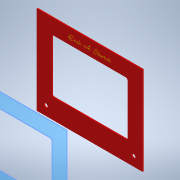
# Autodesk Inventor part: front
Saved by Autodesk Inventor 2022 (Build 260153000, 153)
## iProperties
Created: 2023-08-31
Part Number: front
Material: Generic
Document SubType Name: Modeling
Designer: THK
Density: 1 g/cm^3
Appearance: Red
Author: THK
Autodesk Inventor part; units mm, degrees
ref_plane "YZ Plane" through (0, 0, 0) normal (1, 0, 0) x (0, 1, 0)
ref_plane "XZ Plane" through (0, 0, 0) normal (0, 1, 0) x (-1, 0, 0)
ref_plane "XY Plane" through (0, 0, 0) normal (0, 0, 1) x (1, 0, 0)
sketch "Sketch1" plane through (0, 0, 0) normal (0, 0, 1) x (1, 0, 0)
  line L0 (-264.1156, 220.8859) -> (264.1156, 220.8859)
  line L1 (264.1156, 220.8859) -> (264.1156, -220.8859)
  line L2 (264.1156, -220.8859) -> (-264.1156, -220.8859)
  line L3 (-264.1156, -220.8859) -> (-264.1156, 220.8859)
  line L4 (-264.1156, 220.8859) -> (264.1156, -220.8859) construction
  line L5 (264.1156, 220.8859) -> (-264.1156, -220.8859) construction
  point P0 (0, 0)
  dimension "d0" = 528.2313
  dimension "d1" = 441.7719
  constraints: 12 end point, 2 midpoint, 2 parallel, 1 horizontal, 1 perpendicular
  measures "d0" distance of L1.end L2.end
  measures "d1" distance of L0.end L1.end
extrude "Extrusion1" add sketch "Sketch1" against normal blind 6
sketch "Sketch2" plane through (0, 0, 0) normal (0, 0, 1) x (1, 0, 0)
  line L0 (-181.2094, 146.2703) -> (181.2094, 146.2703)
  line L1 (189.5, 137.9797) -> (189.5, -113.1078)
  line L2 (181.2094, -121.3984) -> (-181.2094, -121.3984)
  line L3 (-189.5, -113.1078) -> (-189.5, 137.9797)
  line L4 (-189.5, 146.2703) -> (189.5, -121.3984) construction
  line L5 (189.5, 146.2703) -> (-189.5, -121.3984) construction
  line L6 (189.5, 105.3059) -> (264.1156, 105.3059) construction
  line L7 (264.1156, 220.8859) -> (264.1156, -220.8859) projected
  line L8 (72.6661, 146.2703) -> (72.6661, 220.8859) construction
  line L9 (-264.1156, 220.8859) -> (264.1156, 220.8859) projected
  arc A0 (-181.2094, 146.2703) -> (-189.5, 137.9797) centre (-181.2094, 137.9797) ccw
  arc A1 (189.5, 137.9797) -> (181.2094, 146.2703) centre (181.2094, 137.9797) ccw
  arc A2 (181.2094, -121.3984) -> (189.5, -113.1078) centre (181.2094, -113.1078) ccw
  arc A3 (-189.5, -113.1078) -> (-181.2094, -121.3984) centre (-181.2094, -113.1078) ccw
  point P0 (0, 0)
  point P1 (0, 12.4359)
  point P2 (0, 12.4359)
  dimension "d4" = 267.6687
  dimension "d5" = 379
  dimension "d6" = 74.6156
  dimension "d7" = 8.2906
  constraints: 16 end point, 12 point on line, 8 point on circle, 8 tangent, 4 centre point, 3 equal radius, 3 midpoint, 2 horizontal, 2 parallel, 2 perpendicular, 1 vertical, 1 vertical alignment
  measures "d4" distance between parallel lines of L2 L0
  measures "d5" distance between parallel lines of L1 L3
  measures "d6" distance between parallel lines of L7 L1
  measures "d7" radius of A0
extrude "Extrusion2" cut sketch "Sketch2" against normal through all
sketch "Sketch3" plane through (0, 0, 0) normal (0, 0, 1) x (1, 0, 0)
  line L0 (-264.1156, -220.8859) -> (-264.1156, 220.8859) construction
  line L1 (-264.1156, -220.8859) -> (-219.1094, -220.8859) construction
  line L2 (-219.1094, -220.8859) -> (-219.1094, -175.8797) construction
  line L3 (-219.1094, -175.8797) -> (-264.1156, -175.8797) construction
  line L4 (-264.1156, -175.8797) -> (-264.1156, -220.8859) construction
  point P0 (0, 0)
  dimension "d10" = 45.0063
  dimension "d11" = 45.0063
  constraints: 8 end point, 2 parallel, 1 coincident, 1 horizontal, 1 perpendicular
  measures "d10" distance of L3.end L2.end
  measures "d11" distance of L2.end L1.end
hole "Hole1" at (-219.1094, -175.8797, 0) direction (0, 0, -1) diameter 19 end through all
mirror "Mirror1" about plane through (0, 0, 0) normal (1, 0, 0) of "Hole1"
sketch "Sketch4" plane through (0, 0, 0) normal (0, 0, 1) x (1, 0, 0)
  line L0 (-128.1015, 195.1507) -> (128.1015, 195.1507) construction
  line L1 (128.1015, 195.1507) -> (128.1015, 162.8739) construction
  line L2 (128.1015, 162.8739) -> (-128.1015, 162.8739) construction
  line L3 (-128.1015, 162.8739) -> (-128.1015, 195.1507) construction
  line L4 (-189.5, 185.6016) -> (189.5, 185.6016) projected
  line L5 (-189.5, -121.3984) -> (-189.5, 185.6016) projected
  line L6 (189.5, -121.3984) -> (-189.5, -121.3984) projected
  line L7 (189.5, 185.6016) -> (189.5, -121.3984) projected
  spline S0 degree 2 poles (-100.767, 183.5729) (-99.0504, 183.5729) (-92.1658, 183.3172) (-90.4492, 183.3172) knots 0 0 0 1 2 2 2
  spline S1 degree 2 poles (-90.4492, 183.3172) (-87.7831, 183.3172) (-86.8335, 183.445) knots 0 0 0 1 1 1
  spline S2 degree 2 poles (-86.8335, 183.445) (-84.7699, 183.7372) (-83.5829, 184.8329) knots 0 0 0 1 1 1
  spline S3 degree 2 poles (-83.5829, 184.8329) (-84.3316, 182.2398) (-87.363, 180.8519) knots 0 0 0 1 1 1
  spline S4 degree 2 poles (-87.363, 180.8519) (-88.5866, 180.2858) (-90.5223, 180.2858) knots 0 0 0 1 1 1
  spline S5 degree 2 poles (-90.5223, 180.2858) (-90.924, 180.2858) (-94.1381, 180.3589) knots 0 0 0 1 1 1
  line L8 (-94.1381, 180.3589) -> (-97.7721, 180.3589)
  spline S6 degree 2 poles (-97.7721, 180.3589) (-98.2286, 180.3589) (-99.9452, 180.2858) knots 0 0 0 1 1 1
  spline S7 degree 2 poles (-99.9452, 180.2858) (-99.7809, 179.2084) (-98.5573, 177.784) knots 0 0 0 1 1 1
  spline S8 degree 2 poles (-98.5573, 177.784) (-96.7129, 175.6291) (-91.0884, 173.0725) (-88.1848, 173.0725) knots 0 0 0 1 2 2 2
  spline S9 degree 2 poles (-88.1848, 173.0725) (-85.9752, 173.0725) (-80.4237, 174.8621) (-78.7619, 176.1404) knots 0 0 0 1 2 2 2
  spline S10 degree 2 poles (-78.7619, 176.1404) (-79.328, 175.0265) (-80.6063, 173.9308) knots 0 0 0 1 1 1
  spline S11 degree 2 poles (-80.6063, 173.9308) (-82.615, 172.2507) (-88.0935, 170.2785) (-90.7779, 170.2785) knots 0 0 0 1 2 2 2
  spline S12 degree 2 poles (-90.7779, 170.2785) (-92.7319, 170.2785) (-97.4069, 171.7942) (-98.8861, 172.9812) knots 0 0 0 1 2 2 2
  spline S13 degree 2 poles (-98.8861, 172.9812) (-100.4931, 174.2595) (-102.8123, 178.3136) (-103.141, 180.3954) knots 0 0 0 1 2 2 2
  spline S14 degree 2 poles (-103.141, 180.3954) (-104.748, 180.3223) (-105.3141, 180.2858) knots 0 0 0 1 1 1
  spline S15 degree 2 poles (-105.3141, 180.2858) (-106.4646, 180.1945) (-107.4142, 179.8658) knots 0 0 0 1 1 1
  spline S16 degree 2 poles (-107.4142, 179.8658) (-106.0993, 182.7328) (-102.8305, 183.4816) knots 0 0 0 1 1 1
  spline S17 degree 2 poles (-102.8305, 183.4816) (-101.8079, 188.3026) (-98.6852, 191.0053) knots 0 0 0 1 1 1
  spline S18 degree 2 poles (-98.6852, 191.0053) (-96.4573, 192.941) (-90.2849, 195.1507) (-87.2717, 195.1507) knots 0 0 0 1 2 2 2
  spline S19 degree 2 poles (-87.2717, 195.1507) (-84.2403, 195.1507) (-81.8298, 194.2559) knots 0 0 0 1 1 1
  spline S20 degree 2 poles (-81.8298, 194.2559) (-78.4697, 193.0506) (-78.4697, 190.5122) knots 0 0 0 1 1 1
  spline S21 degree 2 poles (-78.4697, 190.5122) (-78.4697, 188.4304) (-80.4237, 185.7277) knots 0 0 0 1 1 1
  spline S22 degree 2 poles (-80.4237, 185.7277) (-80.3506, 188.1383) (-82.4872, 190.8957) (-84.8612, 191.6627) knots 0 0 0 1 2 2 2
  spline S23 degree 2 poles (-84.8612, 191.6627) (-86.943, 192.3201) (-89.2805, 192.3201) knots 0 0 0 1 1 1
  spline S24 degree 2 poles (-89.2805, 192.3201) (-91.8736, 192.3201) (-94.7042, 191.3705) knots 0 0 0 1 1 1
  spline S25 degree 2 poles (-94.7042, 191.3705) (-97.8634, 190.3114) (-100.5661, 186.8417) (-100.767, 183.5729) knots 0 0 0 1 2 2 2
  line L9 (-74.2148, 185.9651) -> (-71.7129, 186.4217)
  line L10 (-71.7129, 186.4217) -> (-72.4434, 182.532)
  spline S26 degree 2 poles (-72.4434, 182.532) (-72.3703, 182.532) (-72.1147, 182.532) knots 0 0 0 1 1 1
  spline S27 degree 2 poles (-72.1147, 182.532) (-71.8225, 182.532) (-71.5851, 182.532) knots 0 0 0 1 1 1
  line L11 (-71.5851, 182.532) -> (-70.7268, 182.532)
  spline S28 degree 2 poles (-70.7268, 182.532) (-68.992, 182.532) (-68.5172, 182.4954) knots 0 0 0 1 1 1
  line L12 (-68.5172, 182.4954) -> (-70.3068, 179.7014)
  spline S29 degree 2 poles (-70.3068, 179.7014) (-71.5486, 179.8658) (-72.8269, 179.9023) knots 0 0 0 1 1 1
  spline S30 degree 2 poles (-72.8269, 179.9023) (-73.0643, 178.8431) (-73.0643, 177.7657) knots 0 0 0 1 1 1
  spline S31 degree 2 poles (-73.0643, 177.7657) (-73.0643, 176.6152) (-71.6581, 175.2822) (-70.4711, 175.2822) knots 0 0 0 1 2 2 2
  spline S32 degree 2 poles (-70.4711, 175.2822) (-69.5033, 175.2822) (-68.8276, 175.3917) knots 0 0 0 1 1 1
  line L13 (-68.8276, 175.3917) -> (-71.8773, 173.1456)
  spline S33 degree 2 poles (-71.8773, 173.1456) (-72.279, 172.8534) (-73.466, 172.8534) knots 0 0 0 1 1 1
  spline S34 degree 2 poles (-73.466, 172.8534) (-74.7809, 172.8534) (-75.5113, 173.9125) knots 0 0 0 1 1 1
  spline S35 degree 2 poles (-75.5113, 173.9125) (-76.1322, 174.8256) (-76.1322, 176.2135) knots 0 0 0 1 1 1
  spline S36 degree 2 poles (-76.1322, 176.2135) (-76.1322, 177.4918) (-75.6392, 179.9571) knots 0 0 0 1 1 1
  spline S37 degree 2 poles (-75.6392, 179.9571) (-76.5888, 179.9023) (-77.6114, 179.7014) knots 0 0 0 1 1 1
  line L14 (-77.6114, 179.7014) -> (-76.2966, 182.3676)
  spline S38 degree 2 poles (-76.2966, 182.3676) (-75.9679, 182.4407) (-75.073, 182.532) knots 0 0 0 1 1 1
  spline S39 degree 2 poles (-75.073, 182.532) (-74.8174, 183.5911) (-74.2148, 185.9651) knots 0 0 0 1 1 1
  line L15 (-56.0263, 176.6152) -> (-56.775, 174.9352)
  spline S40 degree 2 poles (-56.775, 174.9352) (-59.6786, 172.8899) (-62.3448, 172.8899) knots 0 0 0 1 1 1
  spline S41 degree 2 poles (-62.3448, 172.8899) (-64.4083, 172.8899) (-67.1476, 175.4648) (-67.1476, 177.4918) knots 0 0 0 1 2 2 2
  spline S42 degree 2 poles (-67.1476, 177.4918) (-67.1476, 179.6284) (-64.7188, 181.2537) knots 0 0 0 1 1 1
  spline S43 degree 2 poles (-64.7188, 181.2537) (-62.5457, 182.6598) (-60.263, 182.6598) knots 0 0 0 1 1 1
  spline S44 degree 2 poles (-60.263, 182.6598) (-57.6698, 182.6598) (-56.2454, 181.2719) knots 0 0 0 1 1 1
  line L16 (-56.2454, 181.2719) -> (-58.4186, 178.2953)
  spline S45 degree 2 poles (-58.4186, 178.2953) (-58.9481, 179.3727) (-61.2308, 180.8884) (-62.3813, 180.8884) knots 0 0 0 1 2 2 2
  spline S46 degree 2 poles (-62.3813, 180.8884) (-64.8466, 180.8884) (-64.8466, 178.8797) knots 0 0 0 1 1 1
  spline S47 degree 2 poles (-64.8466, 178.8797) (-64.8466, 177.4735) (-63.3674, 176.4874) knots 0 0 0 1 1 1
  spline S48 degree 2 poles (-63.3674, 176.4874) (-62.0526, 175.5926) (-60.5734, 175.5926) knots 0 0 0 1 1 1
  spline S49 degree 2 poles (-60.5734, 175.5926) (-58.382, 175.5926) (-56.0263, 176.6152) knots 0 0 0 1 1 1
  line L17 (-51.2235, 190.074) -> (-47.6625, 190.8592)
  spline S50 degree 2 poles (-47.6625, 190.8592) (-49.1235, 186.3486) (-51.0592, 176.9074) knots 0 0 0 1 1 1
  spline S51 degree 2 poles (-51.0592, 176.9074) (-49.8356, 178.4231) (-48.2286, 180.1032) knots 0 0 0 1 1 1
  spline S52 degree 2 poles (-48.2286, 180.1032) (-47.5712, 180.7789) (-46.7129, 181.6372) knots 0 0 0 1 1 1
  spline S53 degree 2 poles (-46.7129, 181.6372) (-45.6538, 182.532) (-44.832, 182.532) knots 0 0 0 1 1 1
  spline S54 degree 2 poles (-44.832, 182.532) (-43.3163, 182.532) (-43.3163, 181.4728) knots 0 0 0 1 1 1
  spline S55 degree 2 poles (-43.3163, 181.4728) (-43.3893, 181.2171) (-43.6267, 179.6649) knots 0 0 0 1 1 1
  spline S56 degree 2 poles (-43.6267, 179.6649) (-43.8824, 177.9849) (-43.8824, 176.5057) knots 0 0 0 1 1 1
  spline S57 degree 2 poles (-43.8824, 176.5057) (-43.8824, 174.6613) (-41.9467, 173.9125) knots 0 0 0 1 1 1
  line L18 (-41.9467, 173.9125) -> (-45.6355, 172.7255)
  spline S58 degree 2 poles (-45.6355, 172.7255) (-47.1147, 173.6751) (-47.1147, 176.2135) knots 0 0 0 1 1 1
  spline S59 degree 2 poles (-47.1147, 176.2135) (-47.1147, 176.4692) (-46.9503, 178.2223) (-46.9503, 178.4597) knots 0 0 0 1 2 2 2
  spline S60 degree 2 poles (-46.9503, 178.4597) (-46.9503, 179.1719) (-47.206, 179.1719) knots 0 0 0 1 1 1
  spline S61 degree 2 poles (-47.206, 179.1719) (-47.6077, 179.1719) (-48.1373, 178.6788) knots 0 0 0 1 1 1
  spline S62 degree 2 poles (-48.1373, 178.6788) (-50.3652, 176.5787) (-52.2827, 173.6021) knots 0 0 0 1 1 1
  line L19 (-52.2827, 173.6021) -> (-54.5836, 172.8534)
  line L20 (-54.5836, 172.8534) -> (-51.2235, 190.074)
  line L21 (4.9123, 194.822) -> (1.7896, 180.7423)
  line L22 (1.7896, 180.7423) -> (4.9123, 180.7423)
  line L23 (4.9123, 180.7423) -> (3.2323, 178.1127)
  line L24 (3.2323, 178.1127) -> (1.187, 178.1127)
  line L25 (1.187, 178.1127) -> (0.2739, 173.9673)
  line L26 (0.2739, 173.9673) -> (-1.9905, 172.8534)
  spline S63 degree 2 poles (-1.9905, 172.8534) (-4.8576, 176.5787) (-9.6056, 178.1127) knots 0 0 0 1 1 1
  spline S64 degree 2 poles (-9.6056, 178.1127) (-10.9204, 176.0857) (-13.0935, 175.0082) knots 0 0 0 1 1 1
  spline S65 degree 2 poles (-13.0935, 175.0082) (-16.3623, 173.4195) (-19.8137, 173.4195) knots 0 0 0 1 1 1
  spline S66 degree 2 poles (-19.8137, 173.4195) (-22.1877, 173.4195) (-25.073, 174.57) knots 0 0 0 1 1 1
  spline S67 degree 2 poles (-25.073, 174.57) (-28.141, 175.7935) (-28.141, 177.9301) knots 0 0 0 1 1 1
  spline S68 degree 2 poles (-28.141, 177.9301) (-28.141, 180.4867) (-25.3835, 182.0024) knots 0 0 0 1 1 1
  spline S69 degree 2 poles (-25.3835, 182.0024) (-23.1008, 183.2259) (-20.3068, 183.2259) knots 0 0 0 1 1 1
  spline S70 degree 2 poles (-20.3068, 183.2259) (-15.9606, 183.2259) (-13.4222, 181.0163) knots 0 0 0 1 1 1
  spline S71 degree 2 poles (-13.4222, 181.0163) (-15.924, 181.3085) (-18.718, 181.3085) knots 0 0 0 1 1 1
  spline S72 degree 2 poles (-18.718, 181.3085) (-22.8999, 181.3085) (-25.1096, 179.9936) knots 0 0 0 1 1 1
  spline S73 degree 2 poles (-25.1096, 179.9936) (-25.7122, 179.6284) (-25.7122, 179.3727) knots 0 0 0 1 1 1
  spline S74 degree 2 poles (-25.7122, 179.3727) (-25.7122, 178.4231) (-23.1008, 177.5283) knots 0 0 0 1 1 1
  spline S75 degree 2 poles (-23.1008, 177.5283) (-19.3207, 176.25) (-16.5267, 176.25) knots 0 0 0 1 1 1
  spline S76 degree 2 poles (-16.5267, 176.25) (-12.0709, 176.25) (-11.5413, 178.1127) knots 0 0 0 1 1 1
  line L27 (-11.5413, 178.1127) -> (-13.55, 178.1127)
  line L28 (-13.55, 178.1127) -> (-11.8517, 180.7423)
  line L29 (-11.8517, 180.7423) -> (-8.7838, 180.7423)
  spline S77 degree 2 poles (-8.7838, 180.7423) (-6.6472, 187.9009) (-4.3645, 190.9688) knots 0 0 0 1 1 1
  spline S78 degree 2 poles (-4.3645, 190.9688) (-2.6297, 193.3428) (-0.2922, 194.128) knots 0 0 0 1 1 1
  spline S79 degree 2 poles (-0.2922, 194.128) (1.3696, 194.6941) (4.9123, 194.822) knots 0 0 0 1 1 1
  line L30 (-7.195, 180.7423) -> (-0.7487, 180.7423)
  line L31 (-0.7487, 180.7423) -> (1.3879, 191.3888)
  spline S80 degree 2 poles (1.3879, 191.3888) (-4.4741, 190.567) (-7.195, 180.7423) knots 0 0 0 1 1 1
  line L32 (-1.8627, 175.1543) -> (-1.2783, 178.1127)
  line L33 (-1.2783, 178.1127) -> (-5.7159, 178.1127)
  line L34 (-5.7159, 178.1127) -> (-3.7436, 176.7431)
  spline S81 degree 2 poles (-3.7436, 176.7431) (-2.9766, 176.2135) (-1.8627, 175.1543) knots 0 0 0 1 1 1
  spline S82 degree 2 poles (21.2381, 180.5963) (20.9825, 179.7927) (20.9825, 179.0805) knots 0 0 0 1 1 1
  spline S83 degree 2 poles (20.9825, 179.0805) (20.9825, 175.9944) (25.1278, 174.57) knots 0 0 0 1 1 1
  spline S84 degree 2 poles (25.1278, 174.57) (28.0131, 173.5838) (31.8481, 173.5838) knots 0 0 0 1 1 1
  spline S85 degree 2 poles (31.8481, 173.5838) (34.8612, 173.5838) (37.1439, 174.2047) knots 0 0 0 1 1 1
  spline S86 degree 2 poles (37.1439, 174.2047) (40.7597, 175.1908) (40.7597, 177.4005) knots 0 0 0 1 1 1
  spline S87 degree 2 poles (40.7597, 177.4005) (40.7597, 178.5875) (39.8649, 179.5736) knots 0 0 0 1 1 1
  spline S88 degree 2 poles (39.8649, 179.5736) (39.0796, 180.4684) (37.8926, 180.8884) knots 0 0 0 1 1 1
  spline S89 degree 2 poles (37.8926, 180.8884) (36.45, 181.3815) (32.6881, 182.6963) knots 0 0 0 1 1 1
  spline S90 degree 2 poles (32.6881, 182.6963) (29.8576, 183.719) (28.5427, 184.6138) knots 0 0 0 1 1 1
  spline S91 degree 2 poles (28.5427, 184.6138) (26.2783, 186.1295) (26.2783, 188.2661) knots 0 0 0 1 1 1
  spline S92 degree 2 poles (26.2783, 188.2661) (26.2783, 190.3114) (28.6158, 192.2288) knots 0 0 0 1 1 1
  spline S93 degree 2 poles (28.6158, 192.2288) (30.5332, 193.7628) (32.8707, 194.4933) knots 0 0 0 1 1 1
  spline S94 degree 2 poles (32.8707, 194.4933) (34.9708, 195.1507) (37.0709, 195.1507) knots 0 0 0 1 1 1
  spline S95 degree 2 poles (37.0709, 195.1507) (40.1023, 195.1507) (42.5676, 193.8906) knots 0 0 0 1 1 1
  spline S96 degree 2 poles (42.5676, 193.8906) (44.4485, 192.941) (44.4485, 191.754) knots 0 0 0 1 1 1
  spline S97 degree 2 poles (44.4485, 191.754) (44.4485, 190.5305) (43.5719, 189.7453) knots 0 0 0 1 1 1
  line L35 (43.5719, 189.7453) -> (40.9606, 187.4443)
  spline S98 degree 2 poles (40.9606, 187.4443) (41.2527, 188.3939) (41.2527, 189.2157) knots 0 0 0 1 1 1
  line L36 (41.2527, 189.2157) -> (41.2527, 189.6722)
  spline S99 degree 2 poles (41.2527, 189.6722) (41.2527, 190.7679) (39.5727, 191.7906) knots 0 0 0 1 1 1
  spline S100 degree 2 poles (39.5727, 191.7906) (37.2352, 193.2332) (34.3681, 193.2332) knots 0 0 0 1 1 1
  spline S101 degree 2 poles (34.3681, 193.2332) (30.6245, 193.2332) (29.2001, 191.1879) knots 0 0 0 1 1 1
  spline S102 degree 2 poles (29.2001, 191.1879) (28.8167, 190.6401) (28.8167, 190.0375) knots 0 0 0 1 1 1
  spline S103 degree 2 poles (28.8167, 190.0375) (28.8167, 188.1565) (31.9394, 186.9513) knots 0 0 0 1 1 1
  spline S104 degree 2 poles (31.9394, 186.9513) (33.3638, 186.4217) (37.0161, 185.0338) knots 0 0 0 1 1 1
  spline S105 degree 2 poles (37.0161, 185.0338) (39.8466, 183.9564) (41.0336, 183.0981) knots 0 0 0 1 1 1
  spline S106 degree 2 poles (41.0336, 183.0981) (43.1702, 181.5459) (43.1702, 179.4458) knots 0 0 0 1 1 1
  spline S107 degree 2 poles (43.1702, 179.4458) (43.1702, 176.7431) (39.9744, 174.4604) knots 0 0 0 1 1 1
  spline S108 degree 2 poles (39.9744, 174.4604) (35.1717, 171.0455) (28.1592, 171.0455) knots 0 0 0 1 1 1
  spline S109 degree 2 poles (28.1592, 171.0455) (23.3747, 171.0455) (20.3798, 173.0177) knots 0 0 0 1 1 1
  spline S110 degree 2 poles (20.3798, 173.0177) (18.2432, 174.4421) (18.2432, 176.2865) knots 0 0 0 1 1 1
  spline S111 degree 2 poles (18.2432, 176.2865) (18.2432, 177.0718) (18.4806, 177.3274) knots 0 0 0 1 1 1
  line L37 (18.4806, 177.3274) -> (21.2381, 180.5963)
  line L38 (47.1695, 190.2018) -> (50.6026, 190.8957)
  spline S112 degree 2 poles (50.6026, 190.8957) (49.5982, 187.4991) (48.393, 179.6284) knots 0 0 0 1 1 1
  spline S113 degree 2 poles (48.393, 179.6284) (51.2783, 183.1346) (53.9445, 183.1346) knots 0 0 0 1 1 1
  spline S114 degree 2 poles (53.9445, 183.1346) (55.1315, 183.1346) (55.9532, 182.605) knots 0 0 0 1 1 1
  spline S115 degree 2 poles (55.9532, 182.605) (56.9576, 182.0206) (56.9576, 180.8884) knots 0 0 0 1 1 1
  spline S116 degree 2 poles (56.9576, 180.8884) (56.9576, 179.5188) (55.2776, 178.3318) knots 0 0 0 1 1 1
  spline S117 degree 2 poles (55.2776, 178.3318) (54.5471, 177.8022) (52.4105, 176.8161) knots 0 0 0 1 1 1
  spline S118 degree 2 poles (52.4105, 176.8161) (54.4193, 175.9944) (57.9072, 175.5196) knots 0 0 0 1 1 1
  line L39 (57.9072, 175.5196) -> (55.1315, 172.7621)
  spline S119 degree 2 poles (55.1315, 172.7621) (51.187, 173.3464) (48.1008, 175.5926) knots 0 0 0 1 1 1
  line L40 (48.1008, 175.5926) -> (49.8722, 177.8935)
  line L41 (49.8722, 177.8935) -> (52.2096, 177.8935)
  spline S120 degree 2 poles (52.2096, 177.8935) (53.3966, 177.8935) (53.3966, 179.1719) knots 0 0 0 1 1 1
  spline S121 degree 2 poles (53.3966, 179.1719) (53.3966, 179.738) (52.5383, 180.6328) (51.9722, 180.6328) knots 0 0 0 1 2 2 2
  spline S122 degree 2 poles (51.9722, 180.6328) (49.8722, 180.6328) (48.6486, 177.9666) knots 0 0 0 1 1 1
  spline S123 degree 2 poles (48.6486, 177.9666) (48.0643, 176.5057) (46.8773, 173.5838) knots 0 0 0 1 1 1
  line L42 (46.8773, 173.5838) -> (44.5033, 172.8534)
  line L43 (44.5033, 172.8534) -> (47.1695, 190.2018)
  line L44 (62.0526, 177.7292) -> (62.6735, 179.2449)
  spline S124 degree 2 poles (62.6735, 179.2449) (64.1527, 178.9527) (65.4675, 178.9527) knots 0 0 0 1 1 1
  spline S125 degree 2 poles (65.4675, 178.9527) (66.0884, 178.9527) (66.0884, 179.5371) knots 0 0 0 1 1 1
  spline S126 degree 2 poles (66.0884, 179.5371) (66.0884, 180.9067) (64.0614, 180.9067) knots 0 0 0 1 1 1
  spline S127 degree 2 poles (64.0614, 180.9067) (61.6143, 180.9067) (61.6143, 178.7153) knots 0 0 0 1 1 1
  spline S128 degree 2 poles (61.6143, 178.7153) (61.6143, 177.7475) (62.5091, 176.9074) knots 0 0 0 1 1 1
  spline S129 degree 2 poles (62.5091, 176.9074) (63.2944, 176.1222) (64.2805, 175.8483) knots 0 0 0 1 1 1
  spline S130 degree 2 poles (64.2805, 175.8483) (64.7736, 175.7204) (65.7049, 175.7204) knots 0 0 0 1 1 1
  spline S131 degree 2 poles (65.7049, 175.7204) (67.6406, 175.7204) (70.3433, 176.7066) knots 0 0 0 1 1 1
  line L45 (70.3433, 176.7066) -> (69.7589, 174.99)
  spline S132 degree 2 poles (69.7589, 174.99) (66.6545, 172.8899) (63.5683, 172.8899) knots 0 0 0 1 1 1
  spline S133 degree 2 poles (63.5683, 172.8899) (61.8152, 172.8899) (59.3134, 175.1908) (59.3134, 176.944) knots 0 0 0 1 2 2 2
  spline S134 degree 2 poles (59.3134, 176.944) (59.3134, 179.1719) (60.5917, 180.5232) knots 0 0 0 1 1 1
  spline S135 degree 2 poles (60.5917, 180.5232) (62.8013, 182.8242) (66.0884, 182.8242) knots 0 0 0 1 1 1
  spline S136 degree 2 poles (66.0884, 182.8242) (67.5128, 182.8242) (68.5719, 182.3311) knots 0 0 0 1 1 1
  spline S137 degree 2 poles (68.5719, 182.3311) (69.9416, 181.6737) (69.9416, 180.4136) knots 0 0 0 1 1 1
  spline S138 degree 2 poles (69.9416, 180.4136) (69.9416, 178.7701) (67.805, 178.0214) knots 0 0 0 1 1 1
  spline S139 degree 2 poles (67.805, 178.0214) (66.3258, 177.4918) (64.2805, 177.4918) knots 0 0 0 1 1 1
  spline S140 degree 2 poles (64.2805, 177.4918) (63.0935, 177.4918) (62.0526, 177.7292) knots 0 0 0 1 1 1
  line L46 (75.1644, 185.9651) -> (77.6662, 186.4217)
  line L47 (77.6662, 186.4217) -> (76.9357, 182.532)
  spline S141 degree 2 poles (76.9357, 182.532) (77.0088, 182.532) (77.2644, 182.532) knots 0 0 0 1 1 1
  spline S142 degree 2 poles (77.2644, 182.532) (77.5566, 182.532) (77.794, 182.532) knots 0 0 0 1 1 1
  line L48 (77.794, 182.532) -> (78.6523, 182.532)
  spline S143 degree 2 poles (78.6523, 182.532) (80.3871, 182.532) (80.8619, 182.4954) knots 0 0 0 1 1 1
  line L49 (80.8619, 182.4954) -> (79.0723, 179.7014)
  spline S144 degree 2 poles (79.0723, 179.7014) (77.8305, 179.8658) (76.5522, 179.9023) knots 0 0 0 1 1 1
  spline S145 degree 2 poles (76.5522, 179.9023) (76.3148, 178.8431) (76.3148, 177.7657) knots 0 0 0 1 1 1
  spline S146 degree 2 poles (76.3148, 177.7657) (76.3148, 176.6152) (77.721, 175.2822) (78.908, 175.2822) knots 0 0 0 1 2 2 2
  spline S147 degree 2 poles (78.908, 175.2822) (79.8758, 175.2822) (80.5515, 175.3917) knots 0 0 0 1 1 1
  line L50 (80.5515, 175.3917) -> (77.5018, 173.1456)
  spline S148 degree 2 poles (77.5018, 173.1456) (77.1001, 172.8534) (75.9131, 172.8534) knots 0 0 0 1 1 1
  spline S149 degree 2 poles (75.9131, 172.8534) (74.5982, 172.8534) (73.8678, 173.9125) knots 0 0 0 1 1 1
  spline S150 degree 2 poles (73.8678, 173.9125) (73.2469, 174.8256) (73.2469, 176.2135) knots 0 0 0 1 1 1
  spline S151 degree 2 poles (73.2469, 176.2135) (73.2469, 177.4918) (73.74, 179.9571) knots 0 0 0 1 1 1
  spline S152 degree 2 poles (73.74, 179.9571) (72.7904, 179.9023) (71.7677, 179.7014) knots 0 0 0 1 1 1
  line L51 (71.7677, 179.7014) -> (73.0825, 182.3676)
  spline S153 degree 2 poles (73.0825, 182.3676) (73.4112, 182.4407) (74.3061, 182.532) knots 0 0 0 1 1 1
  spline S154 degree 2 poles (74.3061, 182.532) (74.5617, 183.5911) (75.1644, 185.9651) knots 0 0 0 1 1 1
  line L52 (93.3528, 176.6152) -> (92.6041, 174.9352)
  spline S155 degree 2 poles (92.6041, 174.9352) (89.7005, 172.8899) (87.0343, 172.8899) knots 0 0 0 1 1 1
  spline S156 degree 2 poles (87.0343, 172.8899) (84.9708, 172.8899) (82.2316, 175.4648) (82.2316, 177.4918) knots 0 0 0 1 2 2 2
  spline S157 degree 2 poles (82.2316, 177.4918) (82.2316, 179.6284) (84.6603, 181.2537) knots 0 0 0 1 1 1
  spline S158 degree 2 poles (84.6603, 181.2537) (86.8335, 182.6598) (89.1161, 182.6598) knots 0 0 0 1 1 1
  spline S159 degree 2 poles (89.1161, 182.6598) (91.7093, 182.6598) (93.1337, 181.2719) knots 0 0 0 1 1 1
  line L53 (93.1337, 181.2719) -> (90.9606, 178.2953)
  spline S160 degree 2 poles (90.9606, 178.2953) (90.431, 179.3727) (88.1483, 180.8884) (86.9978, 180.8884) knots 0 0 0 1 2 2 2
  spline S161 degree 2 poles (86.9978, 180.8884) (84.5325, 180.8884) (84.5325, 178.8797) knots 0 0 0 1 1 1
  spline S162 degree 2 poles (84.5325, 178.8797) (84.5325, 177.4735) (86.0117, 176.4874) knots 0 0 0 1 1 1
  spline S163 degree 2 poles (86.0117, 176.4874) (87.3265, 175.5926) (88.8057, 175.5926) knots 0 0 0 1 1 1
  spline S164 degree 2 poles (88.8057, 175.5926) (90.9971, 175.5926) (93.3528, 176.6152) knots 0 0 0 1 1 1
  line L54 (98.1556, 190.074) -> (101.7166, 190.8592)
  spline S165 degree 2 poles (101.7166, 190.8592) (100.2557, 186.3486) (98.3199, 176.9074) knots 0 0 0 1 1 1
  spline S166 degree 2 poles (98.3199, 176.9074) (99.5435, 178.4231) (101.1505, 180.1032) knots 0 0 0 1 1 1
  spline S167 degree 2 poles (101.1505, 180.1032) (101.8079, 180.7789) (102.6662, 181.6372) knots 0 0 0 1 1 1
  spline S168 degree 2 poles (102.6662, 181.6372) (103.7253, 182.532) (104.5471, 182.532) knots 0 0 0 1 1 1
  spline S169 degree 2 poles (104.5471, 182.532) (106.0628, 182.532) (106.0628, 181.4728) knots 0 0 0 1 1 1
  spline S170 degree 2 poles (106.0628, 181.4728) (105.9898, 181.2171) (105.7524, 179.6649) knots 0 0 0 1 1 1
  spline S171 degree 2 poles (105.7524, 179.6649) (105.4967, 177.9849) (105.4967, 176.5057) knots 0 0 0 1 1 1
  spline S172 degree 2 poles (105.4967, 176.5057) (105.4967, 174.6613) (107.4324, 173.9125) knots 0 0 0 1 1 1
  line L55 (107.4324, 173.9125) -> (103.7436, 172.7255)
  spline S173 degree 2 poles (103.7436, 172.7255) (102.2644, 173.6751) (102.2644, 176.2135) knots 0 0 0 1 1 1
  spline S174 degree 2 poles (102.2644, 176.2135) (102.2644, 176.4692) (102.4288, 178.2223) (102.4288, 178.4597) knots 0 0 0 1 2 2 2
  spline S175 degree 2 poles (102.4288, 178.4597) (102.4288, 179.1719) (102.1731, 179.1719) knots 0 0 0 1 1 1
  spline S176 degree 2 poles (102.1731, 179.1719) (101.7714, 179.1719) (101.2418, 178.6788) knots 0 0 0 1 1 1
  spline S177 degree 2 poles (101.2418, 178.6788) (99.0139, 176.5787) (97.0964, 173.6021) knots 0 0 0 1 1 1
  line L56 (97.0964, 173.6021) -> (94.7955, 172.8534)
  line L57 (94.7955, 172.8534) -> (98.1556, 190.074)
  point P0 (0, 0)
  point P1 (0, 162.8739)
  constraints: 1 midpoint, 1 vertical alignment, 2 other
extrude "Extrusion4" add sketch "Sketch4" along normal blind 2 contours S17 S18 S19 S20 S21 S22 S23 S24 S25 L4 | L4 S25 S0 S1 S2 S3 S4 S5 L8 S6 S7 S8 S9 S10 S11 S12 S13 S14 S15 S16 S17 | S39 L9 L10 L4 | L4 L10 S26 S27 L11 S28 L12 S29 S30 S31 S32 L13 S33 S34 S35 S36 S37 L14 S38 S39 | S165 S166 S167 S168 S169 S170 S171 S172 L55 S173 S174 S175 S176 S177 L56 L57 L4 | L4 L57 L54 S165 | L20 L17 S50 L4 | L4 S50 S51 S52 S53 S54 S55 S56 S57 L18 S58 S59 S60 S61 S62 L19 L20 | L47 S141 S142 L48 S143 L49 S144 S145 S146 S147 L50 S148 S149 S150 S151 S152 L51 S153 S154 L4 | L4 S154 L46 L47 | S77 S78 S79 L21 L4 L31 S80 | L4 S80 L30 L31 L21 L22 L23 L24 L25 L26 S63 S64 S65 S66 S67 S68 S69 S70 S71 S72 S73 S74 S75 S76 L27 L28 L29 S77 | S112 S113 S114 S115 S116 S117 S118 L39 S119 L40 L41 S120 S121 S122 S123 L42 L43 L4 | L4 L43 L38 S112 | S104 S105 S106 S107 S108 S109 S110 S111 L37 S82 S83 S84 S85 S86 S87 S88 S89 S90 S91 L4 | L4 S91 S92 S93 S94 S95 S96 S97 L35 S98 L36 S99 S100 S101 S102 S103 S104 | L15 S40 S41 S42 S43 S44 L16 S45 S46 S47 S48 S49 | L44 S124 S125 S126 S127 S128 S129 S130 S131 L45 S132 S133 S134 S135 S136 S137 S138 S139 S140 | L52 S155 S156 S157 S158 S159 L53 S160 S161 S162 S163 S164
body "Solid1"
